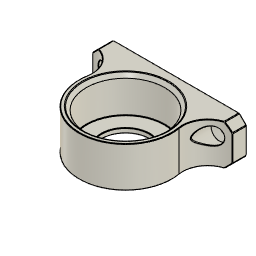
Držák Power CA v8 (Autodesk Fusion 360 design; units mm, degrees)
Autodesk Fusion 360 part; units mm, degrees
sketch "Sketch1" plane through (0, 0, 0) normal (0, 0, 1) x (1, 0, 0)
  circle A0 centre (0, 0) radius 16.5
  circle A1 centre (0, 0) radius 19.5
  line L0 (29.5, 19.5) -> (-29.5, 19.5)
  line L1 (-29.5, 19.5) -> (-29.5, 21.5)
  line L2 (-29.5, 21.5) -> (29.5, 21.5)
  line L3 (29.5, 21.5) -> (29.5, 19.5)
  line L4 (29.5, 19.5) -> (-29.5, 21.5) construction
  line L5 (-29.5, 19.5) -> (29.5, 21.5) construction
  line L6 (-19.5, 0) -> (-19.5, 19.5) construction
  line L7 (-29.5, 19.5) -> (-29.5, 15.5)
  arc A2 (-19.2185, 3.3016) -> (-29.5, 15.5) centre (-29.5, 5.0679) ccw
  line L8 (0, 2.5) -> (0, 20)
  line L9 (29.5, 19.5) -> (29.5, 15.5)
  arc A3 (29.5, 15.5) -> (19.2185, 3.3016) centre (29.5, 5.0679) ccw
  line L10 (-19.2678, -3) -> (-16.225, -3)
  line L11 (16.225, -3) -> (19.2678, -3)
  circle A4 centre (0, 0) radius 10
  point P0 (0, 20.5)
  dimension "d1" = 33
  dimension "d2" = 3
  dimension "d3" = 2
  dimension "d4" = 10
  dimension "d5" = 6
  dimension "d6" = 3
  dimension "d7" = 20
  constraint coincident A0.centre A1.centre
  constraint horizontal L0
  constraint perpendicular L0 L1
  constraint parallel L0 L2
  constraint parallel L1 L3
  constraint coincident L4 P0
  constraint coincident L5 P0
  constraint vertical A0.centre P0
  constraint tangent A1 L0
  constraint coincident A1 L6.start
  constraint coincident L0 L6.end
  constraint perpendicular L0 L6
  constraint tangent A1 L6
  constraint tangent A1 A2
  constraint coincident A1 A2.start
  constraint perpendicular L0 L7
  constraint vertical L0.end A2.centre
  constraint symmetric L0.end L8 L0.start
  constraint symmetric L7.end L8 L9.end
  constraint symmetric A2.start L8 A3.end
  constraint symmetric A2 L8 A3
  constraint coincident A1 L10.start
  constraint coincident A1 L11.end
  constraint horizontal L10
  constraint coincident A0 L10.end
  constraint coincident A0 L11.start
  constraint collinear L10 L11
  constraint concentric A0 A4
  measures "d1" diameter of A0
  measures "d3" distance of L0.end L1.end
  measures "d4" distance of L1 L6
  measures "d5" distance of L1.end L7.end
  measures "d6" distance of A0.centre L10
  measures "d7" diameter of A4
extrude "Extrude1" add sketch "Sketch1" against normal blind 2
extrude "Extrude2" add sketch "Sketch1" along normal blind 15 contours A0 A1 L8 L10 | A0 A1 L10 L11 | A0 A1 L8 L11 | A1 L0 L9 A3 | L0 L1 L2 L3 | A1 L0 L7 A2
sketch "Sketch2" plane through (0, 21.5, 0) normal (0, 1, 0) x (-1, 0, 0)
  line L0 (-29.5, 15) -> (-29.5, -2)
  line L1 (-29.5, -2) -> (29.5, -2)
  line L2 (29.5, -2) -> (29.5, 15)
  line L3 (29.5, 15) -> (-29.5, 15)
  line L4 (19.2185, 15) -> (19.2185, -2)
  line L5 (-19.5, -2) -> (19.5, -2)
  line L6 (-19.2185, -2) -> (-19.2185, 15)
  line L7 (19.5, 15) -> (-19.5, 15)
  line L8 (-19.5, 15) -> (-19.5, -2) construction
  line L9 (-29.5, 6.5) -> (-19.5, 6.5) construction
  circle A0 centre (-23, 9) radius 1.6
  line L10 (0, 20) -> (0, 2.5)
  circle A1 centre (23, 9) radius 1.6
  circle A2 centre (-23, 9) radius 3.5
  circle A3 centre (23, 9) radius 3.5
  point P0 (-29.5, 6.5)
  point P1 (-23, 9)
  dimension "d12" = 3.2
  dimension "d14" = 7
  dimension "d39" = 6
  constraint midpoint L0 P0
  constraint coincident L7.end L8.start
  constraint coincident L5.start L8.end
  constraint coincident P0 L9.start
  constraint midpoint L8 L9.end
  constraint coincident P1 A0.centre
  constraint symmetric A0 L10 A1
  constraint symmetric L10 A2 A3
  constraint tangent L8 A2
  measures "d12" diameter of A0
  measures "d14" diameter of A2
  measures "d39" distance of L3 P1
extrude "Extrude3" cut sketch "Sketch2" against normal through all contours A0 | A1
extrude "Extrude4" cut sketch "Sketch2" against normal blind 15 from surface at -5 contours A2 | A3
chamfer "Chamfer1" distance 1.9 angle 45 2 edges at (-21.5083, 16.5, 9.5786) (24.4917, 16.5, 9.5786)
chamfer "Chamfer2" distance 3 angle 45 4 edges at (-29.5, 18.5, -2) (-29.5, 18.5, 15) (29.5, 18.5, -2) (29.5, 18.5, 15)
chamfer "Chamfer3" distance 1.5 angle 45 1 edges at (-15.3834, 5.9667, 15)
chamfer "Chamfer4" distance 0.2 angle 45 4 edges at (-19.5, 8.0393, 9) (26.5, 15.0593, 9) (-9.3233, 3.6162, 0) (-15.3834, -5.9667, 0) 9 faces at (-7.226, 21.5, 1.3662) (-0.2491, 17.6573, -2) (27.939, 19.4544, -0.561) (29.5, 17.5, 8.3333) (20.0978, 16.1464, 15) (27.939, 19.4544, 13.561) (-28.0505, 19.4708, 13.4495) (-29.5, 17.5, 8.3333) (-28.0505, 19.4708, -0.4495)
named bodies: "Držák Power CA"
